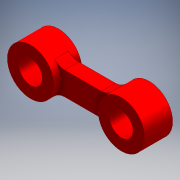
# Autodesk Inventor part: Bielletta
Saved by Autodesk Inventor 2016 (Build 200138000, 138)
## iProperties
Created: 2016-09-10
Part Number: Bielletta
Material: Generic
Document SubType Name: Modeling
Designer: Muhammad
Density: 1 g/cm^3
Appearance: Default
Author: Muhammad
Autodesk Inventor part; units mm, degrees
ref_plane "YZ Plane" through (0, 0, 0) normal (1, 0, 0) x (0, 1, 0)
ref_plane "XZ Plane" through (0, 0, 0) normal (0, 1, 0) x (-1, 0, 0)
ref_plane "XY Plane" through (0, 0, 0) normal (0, 0, 1) x (1, 0, 0)
sketch "Sketch1" plane through (0, 0, 0) normal (0, 1, 0) x (-1, 0, 0)
  circle A0 centre (0, 0) radius 5
  circle A1 centre (0, 0) radius 2.5
  dimension "d1" = 5
  constraints: 2 centre point, 2 coincident
  measures "d1" diameter of A1
extrude "Extrusion1" add sketch "Sketch1" along normal mid plane 6
sketch "Sketch2" plane through (0, 0, 0) normal (0, 1, 0) x (-1, 0, 0)
  point P0 (0, 0)
sketch "Sketch3" plane through (0, 0, 0) normal (0, 1, 0) x (-1, 0, 0)
  circle A0 centre (-19.5, 0) radius 5
  circle A1 centre (-19.5, 0) radius 2.5
  point P0 (0, 0)
  dimension "d5" = 10
  dimension "d6" = 5
  constraints: 2 centre point, 1 coincident
  measures "d5" diameter of A0
  measures "d6" diameter of A1
extrude "Extrusion2" add sketch "Sketch3" along normal mid plane 6
sketch "Sketch4" plane through (0, 0, 0) normal (0, 0, 1) x (1, 0, 0)
  line L0 (3.9419, 0) -> (16.4981, 0) construction
  line L1 (3.9419, 0) -> (3.9419, 1.5)
  line L2 (5, 3) -> (-5, 3) projected
  line L3 (3.9419, 0) -> (3.9419, -1.5)
  line L4 (3.9419, 1.5) -> (16.0281, 1.5)
  line L5 (16.0281, 1.5) -> (16.0281, -1.5)
  line L6 (16.0281, -1.5) -> (3.9419, -1.5)
  line L7 (2.5, -3) -> (2.5, 3) projected
  point P0 (0, 0)
  constraints: 12 end point, 3 perpendicular, 2 horizontal, 1 vertical
extrude "Extrusion3" add sketch "Sketch4" along normal mid plane 5
fillet "Fillet1" radius 3 4 edges at (4.3301, 0, -2.5) (15.1699, 0, -2.5) (15.1699, 0, 2.5) (4.3301, 0, 2.5)
body "Solid1"
